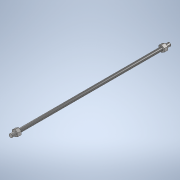
# Autodesk Inventor part: ось пушки 2
Saved by Autodesk Inventor 2020.1 (Build 241239000, 239)
## iProperties
Created: 2022-04-01
Part Number: ось пушки 2
Material: Сталь, литейная
Document SubType Name: Modeling
Designer: User
Density: 7.85 g/cm^3
Appearance: С умеренной полировкой
Author: User
Autodesk Inventor part; units mm, degrees
ref_plane "YZ Plane" through (0, 0, 0) normal (1, 0, 0) x (0, 1, 0)
ref_plane "XZ Plane" through (0, 0, 0) normal (0, 1, 0) x (-1, 0, 0)
ref_plane "XY Plane" through (0, 0, 0) normal (0, 0, 1) x (1, 0, 0)
sketch "Эскиз1" plane through (0, 0, 0) normal (0, 0, 1) x (1, 0, 0)
  circle A0 centre (0, 0) radius 2
  dimension "d0" = 4
  constraints: 1 centre point, 1 coincident
  measures "d0" diameter of A0
extrude "Выдавливание1" add sketch "Эскиз1" along normal blind 83
sketch "Эскиз2" plane through (0, 0, 83) normal (0, 0, 1) x (1, 0, 0)
  line L0 (0, 3.7538) -> (3.2509, 1.8769)
  line L1 (3.2509, 1.8769) -> (3.2509, -1.8769)
  line L2 (3.2509, -1.8769) -> (0, -3.7538)
  line L3 (0, -3.7538) -> (-3.2509, -1.8769)
  line L4 (-3.2509, -1.8769) -> (-3.2509, 1.8769)
  line L5 (-3.2509, 1.8769) -> (0, 3.7538)
  point P0 (0, 0)
  point P1 (0, 0)
  constraints: 12 end point, 1 coincident, 13 other
extrude "Выдавливание2" add sketch "Эскиз2" along normal blind 4
sketch "Эскиз3" plane through (0, 0, 87) normal (0, 0, 1) x (1, 0, 0)
  circle A0 centre (0, 0) radius 2 projected
  circle A1 centre (0, 0) radius 2
  constraints: 1 centre point, 1 coincident
extrude "Выдавливание3" add sketch "Эскиз3" along normal blind 5
thread "Резьба1" size "M4x0.7" class "6g" standard "ANSI Metric M Profile" full length
mirror "Зеркальное отражение1" about plane through (0, 0, 0) normal (0, 0, -1)
